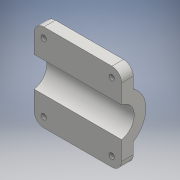
# Autodesk Inventor part: Roof
Saved by Autodesk Inventor 2016 (Build 200138000, 138)
## iProperties
Created: 2017-02-05
Part Number: Roof
Material: PC/ABS Plastic
Document SubType Name: Modeling
Designer: Liquid Metal Printer
Density: 0.357273 g/cm^3
Appearance: Smooth - White
Author: Liquid Metal Printer
Autodesk Inventor part; units mm, degrees
ref_plane "YZ Plane" through (0, 0, 0) normal (1, 0, 0) x (0, 1, 0)
ref_plane "XZ Plane" through (0, 0, 0) normal (0, 1, 0) x (-1, 0, 0)
ref_plane "XY Plane" through (0, 0, 0) normal (0, 0, 1) x (1, 0, 0)
sketch "Sketch1" plane through (0, 0, 0) normal (0, 1, 0) x (-1, 0, 0)
  line L0 (0, 0) -> (-45, 0)
  line L1 (-45, 0) -> (-45, -45)
  line L2 (-45, -45) -> (0, -45)
  line L3 (0, -45) -> (0, 0)
  dimension "d0" = 45
  dimension "d1" = 45
  constraints: 8 end point, 2 parallel, 1 horizontal, 1 perpendicular
  measures "d0" distance of L2.end L1.end
  measures "d1" distance of L1.end L0.end
extrude "Extrusion1" add sketch "Sketch1" along normal blind 6
sketch "Sketch2" plane through (45, 0, 0) normal (1, 0, 0) x (0, 0, -1)
  line L0 (0, 0) -> (45, 0) projected
  line L1 (45, 0) -> (45, 6) projected
  line L2 (0, 6) -> (45, 6) projected
  line L3 (0, 0) -> (0, 6) projected
  line L4 (22.5, 0) -> (30.25, 0)
  line L5 (0, 0) -> (45, 0) projected
  line L6 (30.25, 0) -> (14.75, 0)
  line L7 (22.5, 0) -> (22.5, 6.5)
  arc A0 (30.25, 0) -> (14.75, 0) centre (22.5, -1.3702) ccw
  line L8 (14.75, 0) -> (8.75, 0)
  line L9 (30.25, 0) -> (36.25, 0)
  line L10 (22.5, 6.5) -> (22.5, 12.5)
  arc A1 (36.25, 0) -> (8.75, 0) centre (22.5, -1.3125) ccw
  arc A2 (30.25, 0) -> (14.75, 0) centre (22.5, -1.3702) ccw
  line L11 (14.75, 0) -> (30.25, 0)
  point P0 (22.5, 3)
  dimension "d4" = 7.75
  dimension "d5" = 15.5
  dimension "d6" = 6.5
  dimension "d7" = 6
  dimension "d8" = 6
  dimension "d9" = 6
  constraints: 14 end point, 9 point on circle, 4 point on line, 3 centre point, 1 collinear, 1 concentric, 1 midpoint, 1 perpendicular, 1 vertical
  measures "d4" distance of L4.start L4.end
  measures "d5" distance of L4.end L6.end
  measures "d6" distance of L4.start L7.end
  measures "d7" distance of L6.end L8.end
  measures "d8" distance of L4.end L9.end
  measures "d9" distance of L7.end L10.end
extrude "Extrusion2" add sketch "Sketch2" against normal blind 45 contours A1 L2 A0 L0 | A1 L10 A0 L2 | A1 L2 A0 L10 | A0 L2 A1 L0
sketch "Sketch3" plane through (45, 0, 0) normal (1, 0, 0) x (0, 0, -1)
  line L0 (0, 0) -> (45, 0)
  line L1 (0, 6) -> (45, 6)
  line L2 (22.5, 0) -> (30.25, 0)
  line L3 (0, 0) -> (45, 0)
  line L4 (30.25, 0) -> (14.75, 0)
  line L5 (22.5, 0) -> (22.5, 6.5)
  arc A0 (30.25, 0) -> (14.75, 0) centre (22.5, -1.3702) ccw
  line L6 (14.75, 0) -> (8.75, 0)
  line L7 (30.25, 0) -> (36.25, 0)
  line L8 (22.5, 6.5) -> (22.5, 12.5)
  arc A1 (30.25, 0) -> (14.75, 0) centre (22.5, -1.3702) ccw
  line L9 (14.75, 0) -> (30.25, 0)
  point P0 (22.5, 3)
  point P1 (22.5, -1.3125)
  dimension "d12" = 7.75
  dimension "d13" = 15.5
  dimension "d14" = 6.5
  dimension "d15" = 6
  dimension "d16" = 6
  dimension "d17" = 6
  constraints: 20 end point, 6 point on circle, 4 point on line, 2 centre point, 1 collinear, 1 concentric, 1 midpoint, 1 perpendicular, 1 vertical
  measures "d12" distance of L5.start L4.start
  measures "d13" distance of L4.start L4.end
  measures "d14" distance of L5.start L5.end
  measures "d15" distance of L4.end L6.end
  measures "d16" distance of L4.start L7.end
  measures "d17" distance of L5.end L8.end
extrude "Extrusion3" cut sketch "Sketch3" against normal blind 45
fillet "Fillet1" radius 5 4 edges at (45, 3, 0) (45, 3, -45) (0, 3, 0) (0, 3, -45)
sketch "Sketch4" plane through (0, 6, 0) normal (0, 1, 0) x (1, 0, 0)
  arc A0 (0, 5) -> (5, 0) centre (5, 5) ccw projected
  line L0 (5, 0) -> (40, 0) projected
  arc A1 (40, 0) -> (45, 5) centre (40, 5) ccw projected
  line L1 (45, 5) -> (45, 10.782) projected
  line L2 (45, 10.782) -> (0, 10.782) projected
  line L3 (0, 10.782) -> (0, 5) projected
  line L4 (45, 10.782) -> (0, 10.782) projected
  line L5 (45, 34.218) -> (45, 10.782) projected
  line L6 (0, 34.218) -> (45, 34.218) projected
  line L7 (0, 10.782) -> (0, 34.218) projected
  arc A2 (5, 45) -> (0, 40) centre (5, 40) ccw projected
  line L8 (0, 40) -> (0, 34.218) projected
  line L9 (0, 34.218) -> (45, 34.218) projected
  line L10 (45, 34.218) -> (45, 40) projected
  arc A3 (45, 40) -> (40, 45) centre (40, 40) ccw projected
  line L11 (40, 45) -> (5, 45) projected
  line L12 (5, 5) -> (5, 40)
  line L13 (5, 40) -> (40, 40)
  line L14 (40, 40) -> (40, 5)
  line L15 (40, 5) -> (5, 5)
  circle A4 centre (5, 5) radius 1.375
  circle A5 centre (40, 5) radius 1.375
  circle A6 centre (5, 40) radius 1.375
  circle A7 centre (40, 40) radius 1.375
  point P0 (0, 0)
  dimension "d21" = 2.75
  dimension "d22" = 2.75
  dimension "d23" = 2.75
  dimension "d24" = 2.75
  constraints: 8 end point, 4 centre point, 4 coincident, 3 perpendicular, 1 vertical
  measures "d21" diameter of A4
  measures "d22" diameter of A5
  measures "d23" diameter of A6
  measures "d24" diameter of A7
extrude "Extrusion4" cut sketch "Sketch4" against normal blind 45 contours A4 L15 L12 | L12 L15 A4 | A5 L15 L14 | L14 L15 A5 | A6 L13 L12 | L12 L13 A6 | A7 L13 L14 | L14 L13 A7
sketch "Sketch5" plane through (0, 0, 0) normal (0, -1, 0) x (1, 0, 0)
  line L0 (45, -5) -> (45, -14.75) projected
  line L1 (45, -14.75) -> (45, -30.25) projected
  line L2 (45, -30.25) -> (45, -40) projected
  arc A0 (40, -45) -> (45, -40) centre (40, -40) ccw projected
  circle A1 centre (40, -40) radius 1.375 projected
  circle A2 centre (40, -5) radius 1.375 projected
  arc A3 (45, -5) -> (40, 0) centre (40, -5) ccw projected
  line L3 (5, 0) -> (40, 0) projected
  circle A4 centre (5, -5) radius 1.375 projected
  arc A5 (5, 0) -> (0, -5) centre (5, -5) ccw projected
  line L4 (0, -14.75) -> (0, -5) projected
  line L5 (0, -30.25) -> (0, -14.75) projected
  line L6 (0, -40) -> (0, -30.25) projected
  arc A6 (0, -40) -> (5, -45) centre (5, -40) ccw projected
  line L7 (40, -45) -> (5, -45) projected
  circle A7 centre (5, -40) radius 1.375 projected
  point P0 (0, 0)
body "Solid1"
